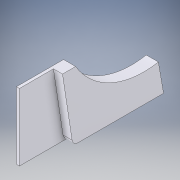
# Autodesk Inventor part: jam-protector-two
Saved by Autodesk Inventor 2019 (Build 230136000, 136)
## iProperties
Created: 2019-05-03
Part Number: jam-protector-two
Material: Generic
Document SubType Name: Modeling
Designer: Tesler
Density: 1 g/cm^3
Appearance: Default
Author: Tesler
## iProperties of the stored document jam-protector-two_3DPrint.ipt
Created: 2019-05-03
Part Number: jam-protector-two_3DPrint
Material: Generic
Document SubType Name: Modeling
Designer: Tesler
Density: 1 g/cm^3
Appearance: Default
Author: Tesler
Autodesk Inventor part; units mm, degrees
ref_plane "YZ Plane" through (0, 0, 0) normal (1, 0, 0) x (0, 1, 0)
ref_plane "XZ Plane" through (0, 0, 0) normal (0, 1, 0) x (-1, 0, 0)
ref_plane "XY Plane" through (0, 0, 0) normal (0, 0, 1) x (1, 0, 0)
sketch "Sketch1" plane through (0, 0, 0) normal (1, 0, 0) x (0, 1, 0)
  line L0 (0, 0.5167) -> (0, -29.5)
  line L1 (0, 0.5167) -> (22.2363, 3.9511)
  line L2 (22.2363, 3.9511) -> (22.2363, -0.3932)
  arc A0 (22.2363, -0.3932) -> (9.8481, -27.7635) centre (35.4748, -22.8739) ccw
  line L3 (0, -29.5) -> (9.8481, -27.7635)
  point P0 (0, 0)
  dimension "d0" = 30.0167
  dimension "d1" = 22.5
  dimension "d2" = 98.78
  dimension "d3" = 9.8481
  dimension "d4" = 80
  dimension "d5" = 26.089
  dimension "d6" = 13.2384
  constraints: 8 end point, 2 point on circle, 2 vertical, 1 centre point
  measures "d0" distance of L0.start L0.end
  measures "d1" distance of L0.start L1.end
  measures "d2" angle of L0 L1
  measures "d3" horizontal distance of L0.end L3.end
  measures "d4" angle of L0 L3
  measures "d5" radius of A0
  measures "d6" distance from line of L2 A0.centre
extrude "Extrusion1" add sketch "Sketch1" along normal blind 3
sketch "Sketch2" plane through (0, 0, 0) normal (-1, 0, 0) x (0, 0, 1)
  line L0 (0.5167, 0) -> (-29.5, 0) projected
  line L1 (3.9511, 22.2363) -> (0.5167, 0) projected
  line L2 (-0.3932, 22.2363) -> (3.9511, 22.2363) projected
  arc A0 (-27.7635, 9.8481) -> (-0.3932, 22.2363) centre (-22.8739, 35.4748) ccw projected
  line L3 (-29.5, 0) -> (-27.7635, 9.8481) projected
  line L4 (3.9511, 22.2363) -> (15.2011, 22.2363)
  line L5 (15.2011, 22.2363) -> (15.2011, 0)
  line L6 (15.2011, 0) -> (-29.5, 0)
  line L7 (0, 0) -> (-29.5, 0) projected
  line L8 (-29.5, 0) -> (-27.7635, 9.8481) projected
  line L9 (-29.5, 0) -> (-27.7635, 9.8481)
  line L10 (3.9511, 22.2363) -> (0.5046, -0.0779) projected
  line L11 (3.9511, 22.2363) -> (-0.3932, 22.2363)
  arc A1 (-27.7635, 9.8481) -> (-0.3932, 22.2363) centre (-22.8739, 35.4748) ccw projected
  arc A2 (-27.7635, 9.8481) -> (-0.3932, 22.2363) centre (-22.8739, 35.4748) ccw
  dimension "d9" = 11.25
  constraints: 10 end point, 2 horizontal, 2 point on circle, 1 centre point, 1 collinear, 1 perpendicular, 1 vertical, 1 other
  measures "d9" distance of L1.start L4.end
extrude "Extrusion2" add sketch "Sketch2" along normal blind 1
fillet "Fillet1" radius 2 1 edges at (1.5, 0, 0.5167)
body "Solid1"
